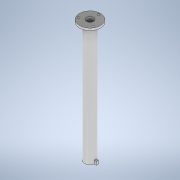
# Autodesk Inventor part: 15
Saved by Autodesk Inventor 2020 (Build 240168000, 168)
## iProperties
Created: 2020-12-23
Part Number: 15
Material: Generic
Document SubType Name: Modeling
Designer: Vikki
Density: 1 g/cm^3
Appearance: Chrome - Polished
Author: Vikki
Autodesk Inventor part; units mm, degrees
ref_plane "XZ Plane" through (0, 0, 0) normal (0, 1, 0) x (-1, 0, 0)
ref_plane "XY Plane" through (0, 0, 0) normal (0, 0, 1) x (1, 0, 0)
sketch "Sketch1" plane through (0, 0, 0) normal (0, 1, 0) x (-1, 0, 0)
  circle A0 centre (0, 0) radius 7.5
  circle A1 centre (0, 0) radius 5
  dimension "d0" = 2.5
  dimension "d1" = 15
  constraints: 2 centre point, 2 coincident
  measures "d0" radial gap between concentric circles of A0 A1
  measures "d1" diameter of A0
extrude "Extrusion1" add sketch "Sketch1" along normal blind 170
ref_plane "Work Plane1" through (7.5, 0, 0) normal (1, 0, 0) x (0, 1, 0)
sketch "Sketch2" plane through (7.5, 0, 0) normal (1, 0, 0) x (0, 1, 0)
  line L0 (0, -7.5) -> (0, 7.5) projected
  line L1 (0, -1.5) -> (0, 1.5)
  line L2 (0, 1.5) -> (5, 1.5)
  line L3 (5, 1.5) -> (5, -1.5)
  line L4 (5, -1.5) -> (0, -1.5)
  point P0 (0, 0)
  dimension "d4" = 1.5
  dimension "d5" = 1.5
  dimension "d6" = 5
  constraints: 8 end point, 2 parallel, 2 point on line, 1 perpendicular
  measures "d4" distance from line of L4 point (0, 0)
  measures "d5" distance from line of L2 point (0, 0)
  measures "d6" distance of L3.end L1.start
extrude "Extrusion2" add sketch "Sketch2" along normal blind 3 and the other way blind 1.5
sketch "Sketch4" plane through (0, 170, 0) normal (0, 1, 0) x (1, 0, 0)
  circle A0 centre (0, 0) radius 15
  circle A1 centre (0, 0) radius 5 projected
  circle A2 centre (0, 12) radius 1.5
  circle A3 centre (-10.3923, -6) radius 1.5
  circle A4 centre (10.3923, -6) radius 1.5
  dimension "d11" = 30
  dimension "d12" = 12
  dimension "d13" = 3
  dimension "d16" = 360
  constraints: 4 centre point, 1 coincident, 1 vertical alignment, 7 other
  measures "d11" diameter of A0
  measures "d12" distance of point (0, 0) A2.centre
  measures "d13" diameter of A2
extrude "Extrusion3" add sketch "Sketch4" along normal blind 3
body "Solid1"
